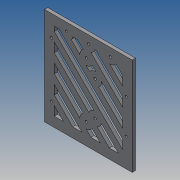
# Autodesk Inventor part: bandeja componentes
Saved by Autodesk Inventor 2017 (Build 210142000, 142)
## iProperties
Part Number: bandeja componentes
Material: Genérico
Document SubType Name: Modeling
Designer: FABLAB
Density: 1 g/cm^3
Appearance: Valor por defecto
Description: Aluminio compuesto routeado CNC
Author: FABLAB
Autodesk Inventor part; units mm, degrees
ref_plane "YZ Plane" through (0, 0, 0) normal (1, 0, 0) x (0, 1, 0)
ref_plane "XZ Plane" through (0, 0, 0) normal (0, 1, 0) x (-1, 0, 0)
ref_plane "XY Plane" through (0, 0, 0) normal (0, 0, 1) x (1, 0, 0)
sketch "Boceto1" plane through (0, 0, 0) normal (0, 1, 0) x (-1, 0, 0)
  line L0 (54, 60) -> (-54, 60)
  line L1 (-54, 60) -> (-54, -60)
  line L2 (-54, -60) -> (54, -60)
  line L3 (54, -60) -> (54, 60)
  line L4 (141.1986, 0) -> (-141.1986, 0) construction
  line L5 (0, -44.0939) -> (0, 44.0939) construction
  point P0 (0, 0)
  point P1 (54, 0)
  point P2 (0, -60)
  point P3 (0, 0)
  dimension "d0" = 108
  dimension "d1" = 120
  constraints: 12 end point, 4 midpoint, 2 horizontal, 2 parallel, 1 coincident, 1 horizontal alignment, 1 perpendicular, 1 vertical, 1 vertical alignment
  measures "d0" distance of L1.end L2.end
  measures "d1" distance of L2.end L0.start
extrude "Extrusión1" add sketch "Boceto1" along normal blind 4
sketch "Boceto2" plane through (0, 4, 0) normal (0, 1, 0) x (1, 0, 0)
  circle A0 centre (-46.5, 36.3333) radius 1.5 projected
  circle A1 centre (-3.5, 36.3333) radius 1.5 projected
  circle A2 centre (-46.5, -31.6667) radius 1.5 projected
  circle A3 centre (-3.5, -31.6667) radius 1.5 projected
  circle A4 centre (4.25, -14.9167) radius 1.5 projected
  circle A5 centre (46.75, -14.9167) radius 1.5 projected
  circle A6 centre (46.75, 23.5833) radius 1.5 projected
  circle A7 centre (4.25, 23.5833) radius 1.5 projected
  circle A8 centre (0, -50) radius 1.5
  circle A9 centre (28, -50) radius 1.5
  circle A10 centre (-28, -50) radius 1.5
  line L0 (-28, -50) -> (28, -50) construction
  line L1 (-54, -60) -> (54, -60) construction
  circle A11 centre (-46.5, 36.3333) radius 7
  circle A12 centre (-3.5, 36.3333) radius 7
  circle A13 centre (4.25, 23.5833) radius 7
  circle A14 centre (46.75, 23.5833) radius 7
  circle A15 centre (46.75, -14.9167) radius 7
  circle A16 centre (4.25, -14.9167) radius 7
  circle A17 centre (-3.5, -31.6667) radius 7
  circle A18 centre (-46.5, -31.6667) radius 7
  circle A19 centre (-28, -50) radius 7
  circle A20 centre (0, -50) radius 7
  circle A21 centre (28, -50) radius 7
  point P0 (0, 0)
  dimension "d9" = 28
  dimension "d10" = 3
  dimension "d11" = 10
  dimension "d33" = 14
  constraints: 14 centre point, 12 coincident, 12 equal radius, 2 end point, 1 horizontal, 1 midpoint, 1 vertical alignment
  measures "d9" distance of L0.end A8.centre
  measures "d10" diameter of A10
  measures "d11" distance between parallel lines of L0 L1
  measures "d33" diameter of A11
sketch "Boceto3" plane through (0, 4, 0) normal (0, 1, 0) x (1, 0, 0)
  line L0 (-54, -60) -> (54, -60) projected
  line L1 (54, -60) -> (54, 60) projected
  line L2 (54, 60) -> (-54, 60) projected
  line L3 (-54, 60) -> (-54, -60) projected
  line L4 (-42, 48) -> (42, 48)
  line L5 (42, 48) -> (42, -48)
  line L6 (42, -48) -> (-42, -48)
  line L7 (-42, -48) -> (-42, 48)
  line L8 (-42, 36.6863) -> (-30.6863, 48)
  line L9 (-42, 25.3726) -> (-19.3726, 48)
  line L10 (-42, 14.0589) -> (-8.0589, 48)
  line L11 (-42, 2.7452) -> (3.2548, 48)
  line L12 (-42, -8.5685) -> (14.5685, 48)
  line L13 (-42, -19.8823) -> (25.8823, 48)
  line L14 (-42, -31.196) -> (37.196, 48)
  line L15 (-42, -42.5097) -> (42, 41.4903)
  line L16 (-36.1766, -48) -> (42, 30.1766)
  line L17 (-24.8629, -48) -> (42, 18.8629)
  line L18 (-13.5492, -48) -> (42, 7.5492)
  line L19 (-2.2355, -48) -> (42, -3.7645)
  line L20 (9.0782, -48) -> (42, -15.0782)
  line L21 (20.3919, -48) -> (42, -26.3919)
  line L22 (31.7056, -48) -> (42, -37.7056)
  point P0 (0, 0)
  point P1 (0, 48)
  point P2 (0, 60)
  dimension "d12" = 12
  dimension "d13" = 12
  dimension "d14" = 12
  dimension "d15" = 45
  dimension "d16" = 8
  dimension "d17" = 8
  dimension "d18" = 8
  dimension "d19" = 8
  dimension "d20" = 8
  dimension "d21" = 8
  dimension "d22" = 8
  dimension "d23" = 8
  dimension "d24" = 8
  dimension "d25" = 8
  dimension "d26" = 8
  dimension "d27" = 8
  dimension "d28" = 8
  dimension "d29" = 8
  dimension "d30" = 8
  constraints: 30 end point, 14 parallel, 1 midpoint, 1 vertical alignment, 43 other
  measures "d15" angle to the sketch x axis of L8
  measures "d16" distance between parallel lines of L8 L9
  measures "d17" distance from line of point (-42, 48) L8
  measures "d18" distance between parallel lines of L9 L10
  measures "d19" distance between parallel lines of L10 L11
  measures "d20" distance between parallel lines of L11 L12
  measures "d21" distance between parallel lines of L12 L13
  measures "d22" distance between parallel lines of L13 L14
  measures "d23" distance between parallel lines of L14 L15
  measures "d24" distance between parallel lines of L15 L16
  measures "d25" distance between parallel lines of L16 L17
  measures "d26" distance between parallel lines of L17 L18
  measures "d27" distance between parallel lines of L18 L19
  measures "d28" distance between parallel lines of L19 L20
  measures "d29" distance between parallel lines of L20 L21
  measures "d30" distance between parallel lines of L21 L22
extrude "Extrusión2" cut sketch "Boceto3" against normal blind 10 contours L4 L8 L7 | L4 L10 L7 L9 | L4 L12 L7 L11 | L4 L14 L7 L13 | L15 L5 L16 L6 L7 | L5 L18 L6 L17 | L5 L20 L6 L19 | L5 L22 L6 L21
extrude "Extrusión3" add sketch "Boceto2" against normal blind 4
sketch "Boceto4" plane through (0, 4, 0) normal (0, 1, 0) x (1, 0, 0)
  circle A0 centre (-46.5, 36.3333) radius 1.5 projected
  circle A1 centre (46.75, 23.5833) radius 1.5 projected
  circle A2 centre (46.75, -14.9167) radius 1.5 projected
  circle A3 centre (28, -50) radius 1.5 projected
  circle A4 centre (0, -50) radius 1.5 projected
  circle A5 centre (-28, -50) radius 1.5 projected
  circle A6 centre (-46.5, -31.6667) radius 1.5 projected
  circle A7 centre (4.25, -14.9167) radius 1.5 projected
  point P0 (0, 0)
extrude "Extrusión4" cut sketch "Boceto4" against normal through all
sketch "Boceto5" plane through (0, 4, 0) normal (0, 1, 0) x (1, 0, 0)
  circle A0 centre (-46.1942, 50) radius 1.5 projected
  circle A1 centre (47.5275, 50) radius 1.5 projected
  circle A2 centre (-46.1942, -50) radius 1.5 projected
  circle A3 centre (47.5275, -50) radius 1.5 projected
  point P0 (0, 0)
extrude "Extrusión5" cut sketch "Boceto5" against normal through all
equation "\"d13\" = d12"
equation "\"d17\" = d16"
equation "\"d18\" = d16"
equation "\"d19\" = d18"
equation "\"d20\" = d19"
equation "\"d21\" = d20"
equation "\"d22\" = d21"
equation "\"d23\" = d22"
equation "\"d24\" = d23"
equation "\"d25\" = d24"
equation "\"d26\" = d25"
equation "\"d27\" = d26"
equation "\"d28\" = d27"
equation "\"d29\" = d28"
equation "\"d30\" = d29"
